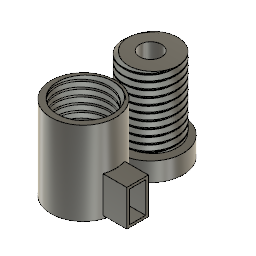
atomizer_redesign v11 (Autodesk Fusion 360 design; units mm, degrees)
Autodesk Fusion 360 part; units mm, degrees
sketch "Sketch1" plane through (0, 0, 0) normal (0, 0, 1) x (1, 0, 0)
  circle A0 centre (0, 0) radius 10
  circle A1 centre (0, 0) radius 12
  circle A2 centre (0, 0) radius 7.5
  dimension "d1" = 20
  dimension "d2" = 24
  dimension "d3" = 15
  constraint coincident A0.centre A1.centre
  constraint concentric A0 A1
  measures "d1" diameter of A0
  measures "d2" diameter of A1
  measures "d3" diameter of A2
extrude "Extrude6" add sketch "Sketch1" along normal blind 1 contours A0 | A1 makes body 1
extrude "Extrude7" add sketch "Sketch1" along normal blind 31 contours A1 bodies 1
sketch "Sketch3" plane through (0, 0, 0) normal (0, 0, 1) x (1, 0, 0)
  line L0 (7.4, -1) -> (7.4, 1)
  line L1 (7.4, -1) -> (11.6, -1)
  line L2 (11.6, -1) -> (11.6, 1)
  line L3 (11.6, 1) -> (7.4, 1)
  dimension "d9" = 2
  constraint vertical L0
  constraint perpendicular L0 L1
  constraint perpendicular L1 L2
  measures "d9" distance of L0.start L0.end
sketch "Sketch4" plane through (0, 0, 0) normal (0, 1, 0) x (1, 0, 0)
sketch "Sketch5" plane through (0, 0, 0) normal (1, 0, 0) x (0, 1, 0)
  line L0 (3.0127, 2.1028, 19.8487) -> (-3.0119, 2.1028, 19.8487)
  line L1 (-3.0119, 2.1028, 19.8487) -> (-3.0119, 13.6628, 19.8487)
  line L2 (-3.0119, 13.6628, 19.8487) -> (3.0127, 13.6628, 19.8487)
  line L3 (3.0127, 13.6628, 19.8487) -> (3.0127, 2.1028, 19.8487)
  line L4 (3.9969, 2.1176, 20.0255) -> (3.9891, 1.1255, 20.15)
  line L5 (-4.0007, 13.6085, 19.9871) -> (-4.0046, 14.5951, 20.15)
  line L6 (-4.0046, 14.5951, 20.15) -> (3.9891, 14.5951, 20.15)
  line L7 (3.9891, 14.5951, 20.15) -> (3.9891, 1.1255, 20.15)
  line L8 (3.9891, 1.1255, 20.15) -> (-4.0046, 1.1255, 20.15)
  line L9 (-4.0046, 1.1255, 20.15) -> (-4.0046, 14.5951, 20.15)
  dimension "d15" = 11.56
  dimension "d19" = 1
  dimension "d20" = 1
  dimension "d22" = 1
  dimension "d23" = 1
extrude "Extrude4" add sketch "Sketch5" against normal blind 9.5 thin wall 1 inside contours L6 L7 L8 L9 in plane through (20.15, 0, 0) normal (1, 0, 0) bodies 1
sketch "Sketch6" plane through (0, 0, 1.1255) normal (0, 0, -1) x (1, 0, 0)
  line L0 (11.3176, -3.9891) -> (20.15, -3.9891)
  line L1 (20.15, -3.9891) -> (20.15, 4.0046)
  line L2 (20.15, 4.0046) -> (11.3121, 4.0046)
  line L3 (12, -1.5) -> (15, -1.5)
  line L4 (15, -1.5) -> (15, 1.5)
  line L5 (15, 1.5) -> (12, 1.5)
  line L6 (12, 1.5) -> (12, -1.5)
  arc A0 (11.3176, -3.9891) -> (11.3121, 4.0046) centre (0, 0) ccw
  dimension "d27" = 3
  dimension "d28" = 3
  constraint horizontal L3
  constraint vertical L4
  constraint horizontal L5
  constraint vertical L6
  measures "d27" distance of L3.start L3.end
  measures "d28" distance of L3.start L5.end
extrude "Extrude5" cut sketch "Sketch6" against normal blind 1 contours L3 L4 L5 L6 bodies 1
extrude "Extrude9" cut sketch "Sketch3" along normal blind 1 bodies 1
thread "Thread3" "ISO Metric profile 22.0 M22x2.5 6H" major diameter 22.2925 minor diameter 19.519 pitch 2.5 angle 60 modelled right hand crest width 0.6905 on face at (-9.9722, 0.7452, 21) from (0, 0, 4) to (0, 0, 31) crest through (9.7595, 0, 1.625) on bodies 1
sketch "Sketch7" plane through (0, 0, 0) normal (0, 0, 1) x (1, 0, 0)
  circle A0 centre (0, 25) radius 12
  circle A1 centre (0, 25) radius 4.05
  circle A2 centre (0, 25) radius 10
  dimension "d45" = 24
  dimension "d48" = 8.1
  dimension "d49" = 20
  constraint concentric A0 A1
  constraint concentric A0 A2
  measures "d45" diameter of A0
  measures "d48" diameter of A1
  measures "d49" diameter of A2
extrude "Extrude10" add sketch "Sketch7" along normal blind 7 separate body contours A0 | A1 | A2 makes body 2
extrude "Extrude12" add sketch "Sketch7" along normal blind 34 contours A2 bodies 2
thread "Thread5" "ISO Metric profile 20.0 M20x2.5 6g" major diameter 19.7905 minor diameter 16.938 pitch 2.5 angle 60 modelled right hand crest width 0.36 on face at (9.9503, 25.9957, 16) crest through (9.8953, 25, 6.375) on bodies 2
sketch "Sketch8" plane through (0, 0, 7) normal (0, 0, 1) x (-1, 0, 0)
  circle A0 centre (0, -25) radius 4.05
  circle A1 centre (0, -25) radius 4.05
  constraint concentric A0 A1
extrude "Extrude13" cut sketch "Sketch8" against normal blind 6 bodies 2
